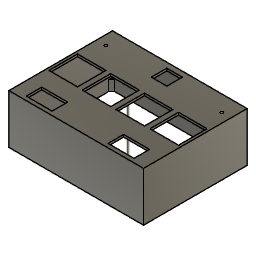
controller_vrch-v5 (Autodesk Fusion 360 design; units mm, degrees)
Autodesk Fusion 360 part; units mm, degrees
sketch "Sketch1" plane through (0, 0, 0) normal (0, 0, 1) x (1, 0, 0)
  line L0 (0, -35) -> (0, -33.2289) construction
  line L1 (0, -33.2289) -> (0, 259.056) construction
  line L2 (-97.9811, 0) -> (484.4158, 0) construction
  line L3 (0, 0) -> (300, 0)
  line L4 (300, 0) -> (300, 200)
  line L5 (300, 200) -> (0, 200)
  line L6 (0, 200) -> (0, 0)
  line L7 (-60, 100) -> (400, 100) construction
  line L8 (25, 100) -> (25, 127.4792)
  line L9 (25, 100) -> (25, 72.5)
  line L10 (25, 127.4792) -> (80, 127.4792)
  line L11 (25, 72.5) -> (80, 72.5)
  line L12 (80, 127.4792) -> (80, 72.5)
  line L13 (21.5, 100) -> (21.5, 131) construction
  line L14 (21.5, 131) -> (83.5, 131) construction
  line L15 (21.4997, 69) -> (83.5, 69) construction
  circle A0 centre (52.5, 100) radius 31 construction
  circle A1 centre (52.5, 100) radius 27.5 construction
  line L16 (83.5, 131) -> (83.5, 69) construction
  line L17 (290, 69) -> (228, 69) construction
  line L18 (290, 100) -> (290, 69) construction
  line L19 (290, 100) -> (290, 131) construction
  line L20 (290, 131) -> (228, 131) construction
  line L21 (228, 131) -> (228, 69) construction
  line L22 (145, 126.7699) -> (90, 126.7699)
  line L23 (146, 151.2972) -> (93.5, 114.6946) construction
  line L24 (93.5, 114.6946) -> (93.5, 69) construction
  line L25 (146, 69) -> (93.5, 69) construction
  line L26 (146, 100) -> (146, 69) construction
  line L27 (146, 100) -> (146, 151.2972) construction
  line L28 (145, 71.7699) -> (90, 71.7699)
  line L29 (90, 126.7699) -> (90, 71.7699)
  line L30 (156, 131) -> (218, 131) construction
  line L31 (218, 131) -> (218, 69) construction
  line L32 (156, 100) -> (156, 131) construction
  line L33 (156, 100) -> (156, 69) construction
  line L34 (156, 69) -> (218, 69) construction
  line L35 (46, 37.5) -> (96, 37.5)
  line L36 (96, 7.5) -> (46, 7.5)
  line L37 (46, 7.5) -> (46, 37.5)
  line L38 (96, 37.5) -> (96, 7.5)
  line L39 (94, 6) -> (44, 6) construction
  line L40 (44, 6) -> (44, 39) construction
  line L41 (44, 39) -> (94, 39) construction
  line L42 (94, 39) -> (94, 6) construction
  line L43 (94, 6) -> (44, 39) construction
  line L44 (44, 6) -> (94, 39) construction
  line L45 (254, 37.5) -> (204, 37.5)
  line L46 (254, 7.5) -> (254, 37.5)
  line L47 (204, 7.5) -> (254, 7.5)
  line L48 (204, 37.5) -> (204, 7.5)
  circle A2 centre (38, 169) radius 2.75
  circle A3 centre (262, 169) radius 2.75
  line L49 (150, 200) -> (150, 0) construction
  line L50 (145, 126.7699) -> (145, 71.7699)
  line L51 (150, 190) -> (135, 190)
  line L52 (150, 190) -> (165, 190)
  line L53 (135, 190) -> (135, 160)
  line L54 (165, 190) -> (165, 160)
  line L55 (165, 160) -> (135, 160)
  line L56 (155, 126.7699) -> (155, 71.7699)
  line L57 (155, 126.7699) -> (210, 126.7699)
  line L58 (155, 71.7699) -> (210, 71.7699)
  line L59 (210, 126.7699) -> (210, 71.7699)
  line L60 (220, 127.4792) -> (220, 72.5)
  line L61 (275, 127.4792) -> (220, 127.4792)
  line L62 (275, 100) -> (275, 127.4792)
  line L63 (275, 100) -> (275, 72.5)
  line L64 (275, 72.5) -> (220, 72.5)
  line L65 (280, 200) -> (280, 0)
  line L66 (20, 200) -> (20, 0)
  point P0 (69, 22.5)
  dimension "d1" = 300
  dimension "d2" = 200
  dimension "d9" = 27.5
  dimension "d12" = 31
  dimension "d13" = 31
  dimension "d14" = 62
  dimension "d15" = 62
  dimension "d17" = 62
  dimension "d18" = 55
  dimension "d31" = 50
  dimension "d32" = 30
  dimension "d37" = 50
  dimension "d38" = 33
  dimension "d39" = 46
  dimension "d40" = 30
  dimension "d41" = 31.5
  dimension "d42" = 5.5
  dimension "d43" = 38
  dimension "d44" = 38
  dimension "d54" = 10
  dimension "d55" = 4
  dimension "d56" = 64
  dimension "d57" = 55
  dimension "d62" = 55
  dimension "d64" = 55
  dimension "d65" = 90
  dimension "d66" = 90
  dimension "d67" = 90
  dimension "d68" = 90
  dimension "d69" = 10
  dimension "d70" = 5
  dimension "d71" = 15
  dimension "d72" = 15
  dimension "d73" = 30
  dimension "d74" = 46
  dimension "d75" = 50
  dimension "d76" = 30
  dimension "d79" = 20
  dimension "d80" = 20
  constraint vertical L0
  constraint parallel L0 L1
  constraint coincident L3.start L1
  constraint horizontal L2
  constraint coincident L3.start L2
  constraint horizontal L3
  constraint vertical L4
  constraint horizontal L5
  constraint vertical L6
  constraint coincident L3.start L6.end
  constraint perpendicular L4 L7
  constraint coincident L7 L8.start
  constraint perpendicular L7 L8
  constraint perpendicular L7 L9
  constraint perpendicular L8 L10
  constraint perpendicular L9 L11
  constraint perpendicular L7 L12
  constraint coincident L7 L13.start
  constraint perpendicular L7 L13
  constraint perpendicular L12 L14
  constraint tangent L13 A0
  constraint tangent L14 A0
  constraint concentric A0 A1
  constraint tangent L8 A1
  constraint tangent L12 A1
  constraint perpendicular L15 L16
  constraint horizontal L35
  constraint horizontal L36
  constraint vertical L37
  constraint perpendicular L36 L38
  constraint horizontal L39
  constraint perpendicular L39 L40
  constraint parallel L39 L41
  constraint parallel L40 L42
  constraint coincident L43 P0
  constraint coincident L44 P0
  constraint midpoint L5 L49.start
  constraint midpoint L3 L49.end
  constraint parallel L29 L49
  constraint parallel L27 L50
  constraint coincident L49 L51.start
  constraint perpendicular L49 L51
  constraint perpendicular L49 L52
  constraint perpendicular L51 L53
  constraint perpendicular L52 L54
  constraint perpendicular L49 L55
  constraint symmetric L8.start L49 L62.start
  constraint symmetric L8.end L49 L61.start
  constraint symmetric L9.end L49 L63.end
  constraint symmetric L10.end L49 L60.start
  constraint symmetric L11.end L49 L60.end
  constraint symmetric L22.start L49 L56.start
  constraint symmetric L22.end L49 L57.end
  constraint symmetric L28.start L49 L56.end
  constraint symmetric L28.end L49 L58.end
  constraint coincident L5 L65.start
  constraint perpendicular L17 L65
  constraint coincident L5 L66.start
  constraint coincident L2 L66.end
  measures "d1" distance of L3.start L3.end
  measures "d2" distance of L3.end L4.end
  measures "d9" distance of L8.start L9.end
  measures "d12" distance of L13.start L13.end
  measures "d13" distance of L13.start L15.start
  measures "d14" distance of L13.end L14.end
  measures "d15" distance of L14.end L15.end
  measures "d17" diameter of A0
  measures "d18" diameter of A1
  measures "d31" distance of L35.start L35.end
  measures "d32" distance of L35.start L36.end
  measures "d37" distance of L40.end L41.end
  measures "d38" distance of L39.end L40.end
  measures "d39" distance of L1 L37
  measures "d40" distance of L15 L41
  measures "d41" distance of L15 L35
  measures "d42" diameter of A2
  measures "d43" distance of L14 A2.centre
  measures "d44" distance of L6 A2.centre
  measures "d54" distance of L16 L24
  measures "d55" distance of L27 L49
  measures "d56" distance of L23.start L23.end
  measures "d57" distance of L22.end L28.end
  measures "d62" horizontal distance of L28.start L28.end
  measures "d64" horizontal distance of L22.start L22.end
  measures "d65" angle of L22 L29
  measures "d66" angle of L28 L29
  measures "d67" angle of L22 L50
  measures "d68" angle of L28 L50
  measures "d69" distance of L12 L29
  measures "d70" distance of L49 L50
  measures "d71" distance of L51.start L51.end
  measures "d72" distance of L51.start L52.end
  measures "d73" distance of L51.end L53.end
  measures "d74" distance of L4 L46
  measures "d75" distance of L45.start L45.end
  measures "d76" distance of L45.end L47.start
  measures "d79" distance of L4 L65
  measures "d80" distance of L1 L66
sketch "Sketch2" plane through (0, 0, 5) normal (0, 0, 1) x (-1, 0, 0)
  line L0 (-145, -71.7699) -> (-90, -71.7699)
  line L1 (-90, -71.7699) -> (-90, -126.7699)
  line L2 (-90, -126.7699) -> (-145, -126.7699)
  circle A0 centre (-38, -169) radius 2.75
  circle A1 centre (-262, -169) radius 2.75
  line L3 (-204, -7.5) -> (-204, -37.5)
  line L4 (-204, -37.5) -> (-254, -37.5)
  line L5 (-254, -37.5) -> (-254, -7.5)
  line L6 (-254, -7.5) -> (-204, -7.5)
  line L7 (-46, -37.5) -> (-96, -37.5)
  line L8 (-96, -37.5) -> (-96, -7.5)
  line L9 (-96, -7.5) -> (-46, -7.5)
  line L10 (-46, -7.5) -> (-46, -37.5)
  line L11 (-25, -72.5) -> (-25, -127.4792)
  line L12 (-25, -127.4792) -> (-80, -127.4792)
  line L13 (-80, -127.4792) -> (-80, -72.5)
  line L14 (-80, -72.5) -> (-25, -72.5)
  line L15 (0, -200) -> (0, 0)
  line L16 (0, 0) -> (-300, 0)
  line L17 (-300, 0) -> (-300, -200)
  line L18 (-300, -200) -> (0, -200)
  line L19 (0, -200) -> (0, 0)
  line L20 (-1, -200) -> (-1, 0)
  line L21 (-299, -200) -> (-299, 0)
  line L22 (-300, -200) -> (-300, 0)
  line L23 (-299, -200) -> (-300, -200)
  line L24 (-300, 0) -> (-299, 0)
  line L25 (-1, 0) -> (0, 0)
  line L26 (0, -200) -> (-1, -200)
  line L27 (-145, -126.7699) -> (-145, -71.7699)
  dimension "d49" = 1
  dimension "d50" = 1
  constraint coincident L15.start L18.end
  constraint coincident L15.end L16.start
  constraint coincident L18 L20.start
  constraint coincident L16 L20.end
  constraint perpendicular L16 L20
  constraint coincident L18 L21.start
  constraint coincident L16 L21.end
  constraint perpendicular L16 L21
  constraint coincident L17.end L18.start
  constraint coincident L16.end L17.start
  measures "d49" distance of L19 L20
  measures "d50" distance of L21 L22
sketch "Sketch5" plane through (0, 0, 0) normal (0, 0, 1) x (1, 0, 0)
  line L0 (20, 200) -> (20, 0)
  line L1 (0, -33.2289) -> (0, 259.056)
  line L2 (280, 200) -> (280, 0)
  line L3 (300, 0) -> (300, 200)
  dimension "d77" = 20
  dimension "d78" = 20
  constraint vertical L0
  constraint vertical L2
  measures "d77" distance of L0 L1
  measures "d78" distance of L2 L3
extrude "Extrude4" add sketch "Sketch1" along normal blind 4.5 contours L3 L5 L65 L66
sketch "Sketch6" plane through (0, 0, 4.5) normal (0, 0, 1) x (-1, 0, 0)
  circle A0 centre (-262, -169) radius 2.75
  line L0 (-90, -71.7699) -> (-90, -126.7699)
  line L1 (-90, -126.7699) -> (-145, -126.7699)
  line L2 (-145, -126.7699) -> (-145, -71.7699)
  line L3 (-145, -71.7699) -> (-90, -71.7699)
  line L4 (-25, -72.5) -> (-25, -127.4792)
  line L5 (-25, -127.4792) -> (-80, -127.4792)
  line L6 (-80, -127.4792) -> (-80, -72.5)
  line L7 (-80, -72.5) -> (-25, -72.5)
  line L8 (-46, -37.5) -> (-96, -37.5)
  line L9 (-96, -37.5) -> (-96, -7.5)
  line L10 (-96, -7.5) -> (-46, -7.5)
  line L11 (-46, -7.5) -> (-46, -37.5)
  line L12 (-204, -7.5) -> (-204, -37.5)
  line L13 (-204, -37.5) -> (-254, -37.5)
  line L14 (-254, -37.5) -> (-254, -7.5)
  line L15 (-254, -7.5) -> (-204, -7.5)
  line L16 (-135, -190) -> (-165, -190)
  line L17 (-165, -190) -> (-165, -160)
  line L18 (-165, -160) -> (-135, -160)
  line L19 (-135, -160) -> (-135, -190)
  circle A1 centre (-38, -169) radius 2.75
  line L20 (-155, -71.7699) -> (-155, -126.7699)
  line L21 (-155, -126.7699) -> (-210, -126.7699)
  line L22 (-210, -126.7699) -> (-210, -71.7699)
  line L23 (-210, -71.7699) -> (-155, -71.7699)
  line L24 (-275, -127.4792) -> (-275, -72.5)
  line L25 (-275, -72.5) -> (-220, -72.5)
  line L26 (-220, -72.5) -> (-220, -127.4792)
  line L27 (-220, -127.4792) -> (-275, -127.4792)
  line L28 (-280, -200) -> (-20, -200)
  line L29 (-20, -200) -> (-20, 0)
  line L30 (-20, 0) -> (-280, 0)
  line L31 (-280, 0) -> (-280, -200)
  line L32 (-23, -200) -> (-23, 0)
  line L33 (-277, -200) -> (-277, 0)
  line L34 (-23, -200) -> (-20, -200)
  line L35 (-20, -200) -> (-20, 0)
  line L36 (-23, 0) -> (-20, 0)
  line L37 (-277, 0) -> (-280, 0)
  line L38 (-280, 0) -> (-280, -200)
  line L39 (-277, -200) -> (-280, -200)
  dimension "d83" = 3
  dimension "d84" = 3
  constraint coincident L28 L32.start
  constraint coincident L30 L32.end
  constraint perpendicular L30 L32
  constraint coincident L28 L33.start
  constraint coincident L30 L33.end
  constraint perpendicular L30 L33
  constraint coincident L28.end L29.start
  constraint coincident L29.end L30.start
  constraint coincident L30.end L31.start
  constraint coincident L28.start L31.end
  measures "d83" distance of L29 L32
  measures "d84" distance of L31 L33
extrude "Extrude5" add sketch "Sketch6" against normal blind 95 contours L28 L30 L31 L33 L37 L38 L39 | L28 L29 L30 L32 L34 L35 L36
sketch "Sketch7" plane through (0, 0, 4.5) normal (0, 0, 1) x (-1, 0, 0)
  line L0 (-20, 0) -> (-280, 0)
  line L1 (-280, 0) -> (-280, -200)
  line L2 (-280, -200) -> (-20, -200)
  line L3 (-20, -200) -> (-20, 0)
  circle A0 centre (-262, -169) radius 2.75
  line L4 (-90, -71.7699) -> (-90, -126.7699)
  line L5 (-90, -126.7699) -> (-145, -126.7699)
  line L6 (-145, -126.7699) -> (-145, -71.7699)
  line L7 (-145, -71.7699) -> (-90, -71.7699)
  line L8 (-25, -72.5) -> (-25, -127.4792)
  line L9 (-25, -127.4792) -> (-80, -127.4792)
  line L10 (-80, -127.4792) -> (-80, -72.5)
  line L11 (-80, -72.5) -> (-25, -72.5)
  line L12 (-46, -37.5) -> (-96, -37.5)
  line L13 (-96, -37.5) -> (-96, -7.5)
  line L14 (-96, -7.5) -> (-46, -7.5)
  line L15 (-46, -7.5) -> (-46, -37.5)
  line L16 (-204, -7.5) -> (-204, -37.5)
  line L17 (-204, -37.5) -> (-254, -37.5)
  line L18 (-254, -37.5) -> (-254, -7.5)
  line L19 (-254, -7.5) -> (-204, -7.5)
  line L20 (-135, -190) -> (-165, -190)
  line L21 (-165, -190) -> (-165, -160)
  line L22 (-165, -160) -> (-135, -160)
  line L23 (-135, -160) -> (-135, -190)
  circle A1 centre (-38, -169) radius 2.75
  line L24 (-155, -71.7699) -> (-155, -126.7699)
  line L25 (-155, -126.7699) -> (-210, -126.7699)
  line L26 (-210, -126.7699) -> (-210, -71.7699)
  line L27 (-210, -71.7699) -> (-155, -71.7699)
  line L28 (-275, -127.4792) -> (-275, -72.5)
  line L29 (-275, -72.5) -> (-220, -72.5)
  line L30 (-220, -72.5) -> (-220, -127.4792)
  line L31 (-220, -127.4792) -> (-275, -127.4792)
  line L32 (-20, -4.5) -> (-280, -4.5)
  line L33 (-20, -195.5) -> (-280, -195.5)
  line L34 (-280, -195.5) -> (-280, -200)
  line L35 (-280, -200) -> (-20, -200)
  line L36 (-20, -195.5) -> (-20, -200)
  line L37 (-20, -4.5) -> (-20, 0)
  line L38 (-20, 0) -> (-280, 0)
  line L39 (-280, 0) -> (-280, -4.5)
  dimension "d87" = 4.5
  dimension "d88" = 4.5
  constraint coincident L3 L32.start
  constraint coincident L1 L32.end
  constraint perpendicular L1 L32
  constraint coincident L3 L33.start
  constraint perpendicular L3 L33
  constraint coincident L1.end L2.start
  constraint perpendicular L2 L34
  constraint coincident L2.end L3.start
  constraint coincident L0.start L3.end
  constraint coincident L0.end L1.start
  measures "d87" distance of L0 L32
  measures "d88" distance of L2 L33
extrude "Extrude6" add sketch "Sketch7" against normal blind 95 contours L0 L1 L3 L32 L37 L38 L39 | L1 L2 L3 L33 L34 L35 L36
sketch "Sketch8" plane through (0, 0, 0) normal (0, 0, -1) x (1, 0, 0)
  line L0 (275, -72.5) -> (275, -127.4792)
  line L1 (275, -127.4792) -> (220, -127.4792)
  line L2 (220, -127.4792) -> (220, -72.5)
  line L3 (220, -72.5) -> (275, -72.5)
  line L4 (155, -126.7699) -> (155, -71.7699)
  line L5 (155, -71.7699) -> (210, -71.7699)
  line L6 (210, -71.7699) -> (210, -126.7699)
  line L7 (210, -126.7699) -> (155, -126.7699)
  circle A0 centre (38, -169) radius 2.75
  line L8 (165, -190) -> (135, -190)
  line L9 (135, -190) -> (135, -160)
  line L10 (135, -160) -> (165, -160)
  line L11 (165, -160) -> (165, -190)
  line L12 (204, -37.5) -> (204, -7.5)
  line L13 (204, -7.5) -> (254, -7.5)
  line L14 (254, -7.5) -> (254, -37.5)
  line L15 (254, -37.5) -> (204, -37.5)
  line L16 (96, -37.5) -> (46, -37.5)
  line L17 (46, -37.5) -> (46, -7.5)
  line L18 (46, -7.5) -> (96, -7.5)
  line L19 (96, -7.5) -> (96, -37.5)
  line L20 (25, -127.4792) -> (25, -72.5)
  line L21 (25, -72.5) -> (80, -72.5)
  line L22 (80, -72.5) -> (80, -127.4792)
  line L23 (80, -127.4792) -> (25, -127.4792)
  line L24 (90, -126.7699) -> (90, -71.7699)
  line L25 (90, -71.7699) -> (145, -71.7699)
  line L26 (145, -71.7699) -> (145, -126.7699)
  line L27 (145, -126.7699) -> (90, -126.7699)
  circle A1 centre (262, -169) radius 2.75
  line L28 (277, -4.5) -> (23, -4.5)
  line L29 (23, -4.5) -> (23, -195.5)
  line L30 (23, -195.5) -> (277, -195.5)
  line L31 (277, -195.5) -> (277, -4.5)
  circle A2 centre (150, -100) radius 2
  circle A3 centre (150, -100) radius 0.5
  dimension "d91" = 1
  constraint concentric A2 A3
  measures "d91" diameter of A3
extrude "Extrude7" add sketch "Sketch8" along normal blind 90 contours A2
sketch "Sketch9" plane through (0, 0, -90.5) normal (0, 0, -1) x (1, 0, 0)
  line L0 (277, -4.5) -> (277, -195.5)
  line L1 (277, -195.5) -> (23, -195.5)
  line L2 (23, -195.5) -> (23, -4.5)
  line L3 (23, -4.5) -> (277, -4.5)
  line L4 (280, 0) -> (20, 0)
  line L5 (20, 0) -> (20, -200)
  line L6 (20, -200) -> (280, -200)
  line L7 (280, -200) -> (280, 0)
  line L8 (271.3431, -4.5) -> (277, -10.1569)
  line L9 (23, -189.8431) -> (28.6569, -195.5)
  line L10 (23, -10.1569) -> (28.6569, -4.5)
  line L11 (277, -189.8431) -> (271.3431, -195.5)
  dimension "d94" = 45
  dimension "d96" = 45
  dimension "d98" = 45
  dimension "d99" = 45
  dimension "d100" = 45
  dimension "d101" = 8
  dimension "d102" = 8
  dimension "d104" = 8
  dimension "d105" = 8
  constraint coincident L3 L8.start
  constraint coincident L0 L8.end
  constraint coincident L2 L9.start
  constraint coincident L1 L9.end
  constraint coincident L2 L10.start
  constraint coincident L3 L10.end
  constraint coincident L0 L11.start
  constraint coincident L1 L11.end
  measures "d94" angle of L3 L8
  measures "d96" angle of L0 L8
  measures "d98" angle of L2 L9
  measures "d99" angle of L3 L10
  measures "d100" angle of L0 L11
  measures "d101" distance of L11.start L11.end
  measures "d102" distance of L9.start L9.end
  measures "d104" distance of L10.start L10.end
  measures "d105" distance of L8.start L8.end
extrude "Extrude8" add sketch "Sketch9" against normal blind 20 contours L0 L3 L8 | L0 L1 L11 | L2 L3 L10 | L1 L2 L9
